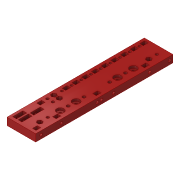
# Autodesk Inventor part: Coupler lift long
Saved by Autodesk Inventor 2020 (Build 240168000, 168)
## iProperties
Created: 2019-10-02
Part Number: Coupler lift long
Material: Generic
Document SubType Name: Modeling
Designer: ball
Density: 1 g/cm^3
Appearance: Default
Author: ball
Autodesk Inventor part; units mm, degrees
sketch "Sketch1" plane through (0, 0, 0) normal (0, 1, 0) x (-1, 0, 0)
  line L0 (0, 0) -> (35.5, 0)
  line L1 (35.5, 0) -> (35.5, -170)
  line L2 (35.5, -170) -> (0, -170)
  line L3 (0, -170) -> (0, 0)
  dimension "d0" = 35.5
  dimension "d1" = 170
  constraints: 8 end point, 2 parallel, 1 horizontal, 1 perpendicular
  measures "d0" distance of L1.end L2.end
  measures "d1" distance of L0.end L1.end
extrude "BlockShape" add sketch "Sketch1" along normal blind 9
sketch "Sketch2" plane through (0, 9, 0) normal (0, 1, 0) x (1, 0, 0)
  circle A0 centre (-10, 15) radius 3.25 construction
  line L0 (-35.5, 0) -> (0, 0) projected
  line L1 (0, 0) -> (0, 170) projected
  line L2 (-13.25, 15) -> (-11.625, 17.8146)
  line L3 (-11.625, 17.8146) -> (-8.375, 17.8146)
  line L4 (-8.375, 17.8146) -> (-6.75, 15)
  line L5 (-6.75, 15) -> (-8.375, 12.1854)
  line L6 (-8.375, 12.1854) -> (-11.625, 12.1854)
  line L7 (-11.625, 12.1854) -> (-13.25, 15)
  circle A1 centre (-10, 150) radius 3.25 construction
  line L8 (-13.25, 150) -> (-11.625, 152.8146)
  line L9 (-11.625, 152.8146) -> (-8.375, 152.8146)
  line L10 (-8.375, 152.8146) -> (-6.75, 150)
  line L11 (-6.75, 150) -> (-8.375, 147.1854)
  line L12 (-8.375, 147.1854) -> (-11.625, 147.1854)
  line L13 (-11.625, 147.1854) -> (-13.25, 150)
  line L14 (0, 170) -> (-35.5, 170) projected
  circle A2 centre (-10, 15) radius 1.7 construction
  circle A3 centre (-10, 150) radius 1.7 construction
  dimension "d7" = 6.5
  dimension "d10" = 6.5
  dimension "d23" = 135
  dimension "d24" = 15
  dimension "d25" = 10
  dimension "d28" = 3.4
  dimension "d29" = 3.4
  constraints: 24 end point, 4 coincident, 2 centre point, 2 horizontal alignment, 30 other
  measures "d23" distance of point (-10, 150) point (-10, 15)
  measures "d24" distance from line of L0 point (-10, 15)
  measures "d25" distance from line of L1 point (-10, 15)
  measures "d28" diameter of A2
  measures "d29" diameter of A3
extrude "SlideNutWell2" cut sketch "Sketch2" against normal blind 5
sketch "Sketch3" plane through (0, 0, 0) normal (0, -1, 0) x (1, 0, 0)
  circle A0 centre (-10, -25) radius 3.25 construction
  line L0 (0, 0) -> (-35.5, 0) projected
  line L1 (-35.5, 0) -> (-35.5, -170) projected
  line L2 (-11.6286, -27.8125) -> (-13.25, -24.9958)
  line L3 (-13.25, -24.9958) -> (-11.6214, -22.1833)
  line L4 (-11.6214, -22.1833) -> (-8.3714, -22.1875)
  line L5 (-8.3714, -22.1875) -> (-6.75, -25.0042)
  line L6 (-6.75, -25.0042) -> (-8.3786, -27.8167)
  line L7 (-8.3786, -27.8167) -> (-11.6286, -27.8125)
  circle A1 centre (-10, -160) radius 3.25 construction
  line L8 (-6.75, -160) -> (-8.375, -162.8146)
  line L9 (-8.375, -162.8146) -> (-11.625, -162.8146)
  line L10 (-11.625, -162.8146) -> (-13.25, -160)
  line L11 (-13.25, -160) -> (-11.625, -157.1854)
  line L12 (-11.625, -157.1854) -> (-8.375, -157.1854)
  line L13 (-8.375, -157.1854) -> (-6.75, -160)
  line L14 (0, -170) -> (0, 0) projected
  dimension "d15" = 6.5
  dimension "d18" = 6.5
  dimension "d16" = 25
  dimension "d19" = 135
  dimension "d26" = 10
  dimension "d27" = 10
  constraints: 24 end point, 2 coincident, 1 horizontal alignment, 31 other
  measures "d16" distance from line of L0 point (-10, -25)
  measures "d19" distance of point (-10, -160) point (-10, -25)
  measures "d26" distance from line of L14 point (-10, -25)
  measures "d27" distance from line of L14 point (-10, -160)
extrude "SlideNutWell1" cut sketch "Sketch3" against normal blind 5
sketch "Sketch5" plane through (0, 9, 0) normal (0, 1, 0) x (1, 0, 0)
  circle A0 centre (-10, 15) radius 1.7
  line L0 (0, 0) -> (0, 170) projected
  line L1 (-35.5, 0) -> (0, 0) projected
  circle A1 centre (-10, 150) radius 1.7
  circle A2 centre (-10, 25) radius 1.7
  circle A3 centre (-10, 160) radius 1.7
  dimension "d30" = 3.4
  dimension "d31" = 10
  dimension "d32" = 15
  dimension "d33" = 3.4
  dimension "d34" = 10
  dimension "d35" = 135
  dimension "d36" = 3.4
  dimension "d37" = 25
  dimension "d38" = 3.4
  dimension "d39" = 10
  dimension "d40" = 135
  constraints: 4 centre point
  measures "d30" diameter of A0
  measures "d31" distance from line of L0 A0.centre
  measures "d32" distance from line of L1 A0.centre
  measures "d33" diameter of A1
  measures "d34" distance from line of L0 A1.centre
  measures "d35" distance of A1.centre A0.centre
  measures "d36" diameter of A2
  measures "d37" distance from line of L1 A2.centre
  measures "d38" diameter of A3
  measures "d39" distance from line of L0 A3.centre
  measures "d40" distance of A2.centre A3.centre
extrude "SlideMoutingHoles" cut sketch "Sketch5" against normal through all
sketch "Sketch6" plane through (0, 9, 0) normal (0, 1, 0) x (1, 0, 0)
  line L0 (-32.5, 4) -> (-27.7502, 4)
  line L1 (-27.7502, 4) -> (-27.7502, 16.7)
  line L2 (-27.7502, 16.7) -> (-32.5, 16.7)
  line L3 (-32.5, 16.7) -> (-32.5, 4)
  line L4 (-35.5, 0) -> (0, 0) projected
  line L5 (-35.5, 170) -> (-35.5, 0) projected
  line L6 (-25.7502, 4) -> (-21.0002, 4)
  line L7 (-21.0002, 4) -> (-21.0002, 16.7)
  line L8 (-21.0002, 16.7) -> (-25.7502, 16.7)
  line L9 (-25.7502, 16.7) -> (-25.7502, 4)
  line L10 (0, 0) -> (0, 170) construction
  line L11 (-35.5, 170) -> (0, 170) projected
  line L12 (0, 0) -> (-20, 0) construction
  line L13 (-20, 0) -> (-20, 170) construction
  line L14 (-20, 170) -> (0, 170) construction
  line L15 (0, 170) -> (0, 0)
  circle A0 centre (-23.3752, 44.7) radius 1.7
  circle A1 centre (-30.125, 44.7) radius 1.7
  circle A2 centre (-30.125, 52.7) radius 1.7
  circle A3 centre (-23.3752, 52.7) radius 1.7
  line L16 (-25.7502, 18.7) -> (-21.0002, 18.7)
  line L17 (-21.0002, 18.7) -> (-21.0002, 31.4)
  line L18 (-21.0002, 31.4) -> (-25.7502, 31.4)
  line L19 (-25.7502, 31.4) -> (-25.7502, 18.7)
  dimension "d43" = 4.7498
  dimension "d44" = 12.7
  dimension "d45" = 4
  dimension "d46" = 3
  dimension "d47" = 4.75
  dimension "d48" = 2
  dimension "d49" = 20
  dimension "d50" = 3.4
  dimension "d51" = 28
  dimension "d87" = 3.4
  dimension "d88" = 5.375
  dimension "d90" = 3.4
  dimension "d91" = 8
  dimension "d92" = 3.4
  dimension "d180" = 4.75
  dimension "d181" = 12.7
  dimension "d182" = 2
  dimension "d183" = 12.7
  dimension "d184" = 4
  dimension "d260" = 28
  dimension "d261" = 8
  constraints: 32 end point, 8 parallel, 4 centre point, 4 horizontal, 4 perpendicular, 2 point on line
  measures "d43" distance of L2.end L1.end
  measures "d44" distance of L1.end L0.end
  measures "d45" distance between parallel lines of L4 L0
  measures "d46" distance between parallel lines of L5 L3
  measures "d47" distance of L8.end L7.end
  measures "d48" distance between parallel lines of L9 L1
  measures "d49" distance of L13.end L14.end
  measures "d50" diameter of A0
  measures "d51" distance from line of A0.centre L8
  measures "d87" diameter of A1
  measures "d88" distance from line of L5 A1.centre
  measures "d90" diameter of A2
  measures "d91" distance of A2.centre A1.centre
  measures "d92" diameter of A3
  measures "d180" distance of L18.end L17.end
  measures "d181" distance of L17.end L16.end
  measures "d182" distance between parallel lines of L16 L8
  measures "d183" distance between parallel lines of L8 L6
  measures "d184" distance between parallel lines of L4 L6
  measures "d260" distance from line of L2 A1.centre
  measures "d261" distance of A0.centre A3.centre
extrude "PulleyHoles" cut sketch "Sketch6" against normal through all contours L3 L2 L1 L0 | L9 L8 L7 L6 | A0 | A1 | A2 | A3 | L19 L18 L17 L16
sketch "Sketch7" plane through (0, 0, 0) normal (0, -1, 0) x (1, 0, 0)
  circle A0 centre (-23.3752, -44.7) radius 1.7 projected
  circle A1 centre (-23.3752, -44.7) radius 3.25 construction
  circle A2 centre (-30.1625, -44.7) radius 3.25 construction
  line L0 (-30.125, -41.4502) -> (-27.3294, -43.1076)
  line L1 (-27.3294, -43.1076) -> (-27.3669, -46.3574)
  line L2 (-27.3669, -46.3574) -> (-30.2, -47.9498)
  line L3 (-30.2, -47.9498) -> (-32.9956, -46.2924)
  line L4 (-32.9956, -46.2924) -> (-32.9581, -43.0426)
  line L5 (-32.9581, -43.0426) -> (-30.125, -41.4502)
  circle A3 centre (-30.125, -44.7) radius 1.7 projected
  line L6 (-20.1252, -44.7) -> (-21.7502, -47.5146)
  line L7 (-21.7502, -47.5146) -> (-25.0002, -47.5146)
  line L8 (-25.0002, -47.5146) -> (-26.6252, -44.7)
  line L9 (-26.6252, -44.7) -> (-25.0002, -41.8854)
  line L10 (-25.0002, -41.8854) -> (-21.7502, -41.8854)
  line L11 (-21.7502, -41.8854) -> (-20.1252, -44.7)
  point P0 (0, 0)
  dimension "d54" = 6.5
  dimension "d89" = 6.5
  dimension "d262" = 0
  constraints: 24 end point, 4 coincident, 1 horizontal alignment, 32 other
  measures "d262" vertical distance of point (-30.162, -44.7) A3.centre
extrude "TensionNutWells2" cut sketch "Sketch7" against normal blind 5 contours A0 | L0 L1 L2 L3 L4 L5 | A3 | L6 L7 L8 L9 L10 L11
sketch "Sketch8" plane through (-35.5, 0, -170) normal (-1, 0, 0) x (0, 0, 1)
  circle A0 centre (159.65, 4.5) radius 1.4605
  line L0 (0, 9) -> (170, 9) projected
  line L1 (170, 0) -> (170, 9) projected
  circle A1 centre (144.95, 4.5) radius 1.45
  dimension "d57" = 2.921
  dimension "d58" = 4.5
  dimension "d59" = 10.35
  dimension "d185" = 2.9
  dimension "d186" = 14.7
  dimension "d187" = 4.5
  constraints: 2 centre point
  measures "d57" diameter of A0
  measures "d58" distance from line of L0 A0.centre
  measures "d59" distance from line of L1 A0.centre
  measures "d185" diameter of A1
  measures "d186" distance of A1.centre A0.centre
  measures "d187" distance from line of L0 A1.centre
hole "PulleyMountingHole" at (-35.5, 4.5, -10.35) at (-35.5, 4.5, -25.05) direction (1, 0, 0) diameter 2.921 depth 21 counterbore diameter 3.4 counterbore depth 1.5
sketch "Sketch9" plane through (-21.0002, 9, -16.7) normal (-1, 0, 0) x (0, 0, 1)
  circle A0 centre (6.35, -4.5) radius 1.4605 projected
  circle A1 centre (6.35, -4.5) radius 2.54
  circle A2 centre (-8.35, -4.5) radius 1.4605 projected
  circle A3 centre (-8.35, -4.5) radius 2.54
  point P0 (16.7, -9)
  dimension "d67" = 5.08
  dimension "d194" = 5.08
  constraints: 2 centre point, 2 coincident
  measures "d67" diameter of A1
  measures "d194" diameter of A3
extrude "PulleyStandoff4" add sketch "Sketch9" along normal blind 0.2032
sketch "Sketch11" plane through (-25.7502, 9, -4) normal (1, 0, 0) x (0, 0, -1)
  circle A0 centre (6.35, -4.5) radius 2.54
  circle A1 centre (6.35, -4.5) radius 1.4605
  circle A2 centre (21.05, -4.5) radius 1.4605 projected
  circle A3 centre (21.05, -4.5) radius 2.54
  point P0 (-4, -9)
  dimension "d73" = 5.08
  dimension "d195" = 5.08
  constraints: 3 centre point, 3 coincident
  measures "d73" diameter of A0
  measures "d195" diameter of A3
sketch "Sketch12" plane through (-32.5, 9, -4) normal (1, 0, 0) x (0, 0, -1)
  circle A0 centre (6.35, -4.5) radius 2.54
  circle A1 centre (6.35, -4.5) radius 1.4605
  point P0 (-4, -9)
  dimension "d76" = 5.08
  constraints: 2 centre point, 1 coincident
  measures "d76" diameter of A0
extrude "PulleyStandoff1" add sketch "Sketch12" along normal blind 0.2032
sketch "Sketch10" plane through (-27.7502, 9, -16.7) normal (-1, 0, 0) x (0, 0, 1)
  circle A0 centre (6.35, -4.5) radius 2.54
  circle A1 centre (6.35, -4.5) radius 1.4605
  point P0 (16.7, -9)
  dimension "d70" = 5.08
  constraints: 2 centre point, 2 coincident
  measures "d70" diameter of A0
extrude "PulleyStandoff2" add sketch "Sketch10" along normal blind 0.2032
extrude "PulleyStandoff3" add sketch "Sketch11" along normal blind 0.2032
sketch "Sketch14" plane through (0, 0, -170) normal (0, 0, -1) x (-1, 0, 0)
  circle A0 centre (18, 4.5) radius 2.25
  line L0 (35.5, 0) -> (0, 0) projected
  line L1 (0, 0) -> (0, 9) projected
  dimension "d82" = 4.5
  dimension "d83" = 4.5
  dimension "d84" = 18
  constraints: 1 centre point
  measures "d82" diameter of A0
  measures "d83" distance from line of L0 A0.centre
  measures "d84" distance from line of L1 A0.centre
extrude "4mmShaftHole" cut sketch "Sketch14" against normal blind 71
sketch "Sketch15" plane through (0, 9, 0) normal (0, 1, 0) x (1, 0, 0)
  circle A0 centre (-30.125, 52.7) radius 1.7 projected
  circle A1 centre (-30.125, 52.7) radius 3.25 construction
  circle A2 centre (-23.3752, 52.7) radius 1.7 projected
  circle A3 centre (-23.3752, 52.7) radius 3.25 construction
  line L0 (-30.125, 49.45) -> (-32.9396, 51.075)
  line L1 (-32.9396, 51.075) -> (-32.9396, 54.325)
  line L2 (-32.9396, 54.325) -> (-30.125, 55.95)
  line L3 (-30.125, 55.95) -> (-27.3104, 54.325)
  line L4 (-27.3104, 54.325) -> (-27.3104, 51.075)
  line L5 (-27.3104, 51.075) -> (-30.125, 49.45)
  line L6 (-23.3752, 49.45) -> (-26.1898, 51.075)
  line L7 (-26.1898, 51.075) -> (-26.1898, 54.325)
  line L8 (-26.1898, 54.325) -> (-23.3752, 55.95)
  line L9 (-23.3752, 55.95) -> (-20.5606, 54.325)
  line L10 (-20.5606, 54.325) -> (-20.5606, 51.075)
  line L11 (-20.5606, 51.075) -> (-23.3752, 49.45)
  point P0 (0, 0)
  dimension "d93" = 6.5
  dimension "d94" = 6.5
  constraints: 24 end point, 4 coincident, 2 vertical alignment, 30 other
extrude "TensionNutWells1" cut sketch "Sketch15" against normal blind 5
ref_plane "PulleyMidPlane1" through (-30.1251, 9, -4) normal (1, 0, 0) x (0, 0, -1)
ref_plane "PulleyMidPlane2" through (-23.3752, 9, -16.7) normal (-1, 0, 0) x (0, 0, 1)
sketch "Sketch16" plane through (0, 9, 0) normal (0, 1, 0) x (1, 0, 0)
  circle A0 centre (-9.525, 40) radius 1.9304 construction
  line L0 (0, 0) -> (0, 170) construction
  circle A1 centre (-10, 25) radius 1.7 construction
  circle A2 centre (-9.525, 59.558) radius 1.9304 construction
  circle A3 centre (-9.525, 130.442) radius 1.9304 construction
  circle A4 centre (-10, 150) radius 1.7 construction
  circle A5 centre (-9.525, 110.884) radius 1.9304 construction
  dimension "d97" = 3.8608
  dimension "d98" = 9.525
  dimension "d99" = 15
  dimension "d100" = 3.8608
  dimension "d101" = 19.558
  dimension "d102" = 3.8608
  dimension "d103" = 9.525
  dimension "d104" = 19.558
  dimension "d105" = 3.8608
  dimension "d106" = 19.558
  constraints: 4 centre point
  measures "d97" diameter of A0
  measures "d98" distance from line of L0 A0.centre
  measures "d99" vertical distance of A1.centre A0.centre
  measures "d100" diameter of A2
  measures "d101" distance of A2.centre A0.centre
  measures "d102" diameter of A3
  measures "d103" distance from line of L0 A3.centre
  measures "d104" vertical distance of A4.centre A3.centre
  measures "d105" diameter of A5
  measures "d106" distance of A3.centre A5.centre
hole "XRailMoutingHoles1" at (-9.525, 9, -40) at (-9.525, 9, -59.558) at (-9.525, 9, -110.884) at (-9.525, 9, -130.442) direction (0, -1, 0) diameter 3.8608 end through all counterbore diameter 8.89 counterbore depth 3.048
sketch "Sketch17" plane through (0, 0, 0) normal (0, -1, 0) x (1, 0, 0)
  circle A0 centre (-9.525, -120.663) radius 1.9304 construction
  circle A1 centre (-9.525, -130.442) radius 1.9304 projected
  circle A2 centre (-9.525, -101.105) radius 1.9304 construction
  circle A3 centre (-9.525, -49.779) radius 1.9304 construction
  circle A4 centre (-9.525, -69.337) radius 1.9304 construction
  circle A5 centre (-9.525, -40) radius 1.9304 construction
  point P0 (0, 0)
  dimension "d114" = 3.8608
  dimension "d115" = 9.779
  dimension "d116" = 3.8608
  dimension "d117" = 19.558
  dimension "d118" = 3.8608
  dimension "d119" = 3.8608
  dimension "d120" = 9.779
  dimension "d121" = 19.558
  constraints: 4 centre point
  measures "d114" diameter of A0
  measures "d115" distance of A0.centre A1.centre
  measures "d116" diameter of A2
  measures "d117" distance of A2.centre A0.centre
  measures "d118" diameter of A3
  measures "d119" diameter of A4
  measures "d120" distance of A3.centre A5.centre
  measures "d121" distance of A4.centre A3.centre
hole "XRailMoutingHoles2" at (-9.525, 0, -120.663) at (-9.525, 0, -101.105) at (-9.525, 0, -69.337) at (-9.525, 0, -49.779) direction (0, 1, 0) diameter 3.8608 end through all counterbore diameter 8.89 counterbore depth 3.048
sketch "Sketch19" plane through (0, 0, 0) normal (1, 0, 0) x (0, 0, -1)
  line L0 (12.1854, 9) -> (12.1854, 4) construction
  line L1 (67.4066, 9) -> (71.2674, 9) construction
  line L2 (99.1746, 9) -> (103.0354, 9) construction
  line L3 (125.997, 9) -> (134.887, 9) construction
  line L4 (147.1854, 9) -> (147.1854, 4) construction
  line L5 (158.3, 9) -> (161.7, 9) construction
  line L6 (170, 0) -> (0, 0) projected
  line L7 (0, 0) -> (0, 9) projected
  circle A0 centre (76.2674, 4.5) radius 1.7
  circle A1 centre (86.2674, 4.5) radius 1.7
  circle A2 centre (96.2674, 4.5) radius 1.7
  line L8 (170, 0) -> (170, 9) projected
  circle A3 centre (165.85, 4.5) radius 1.7
  dimension "d159" = 27.9072
  dimension "d160" = 3.4
  dimension "d161" = 4.5
  dimension "d162" = 5
  dimension "d165" = 10
  dimension "d170" = 8.3
  dimension "d171" = 3.4
  dimension "d172" = 4.5
  dimension "d173" = 4.15
  dimension "d174" = 12.2984
  constraints: 4 centre point, 1 horizontal, 4 other
  measures "d159" distance of L1.end L2.start
  measures "d160" diameter of A0
  measures "d161" distance from line of L6 A0.centre
  measures "d162" horizontal distance of L1.end A0.centre
  measures "d165" distance of A0.centre A1.centre
  measures "d170" distance from line of L8 L5.end
  measures "d171" diameter of A3
  measures "d172" distance from line of L6 A3.centre
  measures "d173" distance from line of L8 A3.centre
  measures "d174" distance from line of L3.end L4
extrude "NonPulleySideHoles" cut sketch "Sketch19" against normal blind 13 contours A0 | A2 | A3
ref_plane "Work Plane3" through (-7.7, 0, 0) normal (1, 0, 0) x (0, 0, -1)
sketch "Sketch20" plane through (-7.7, 0, 0) normal (1, 0, 0) x (0, 0, -1)
  circle A0 centre (6.65, 4.5) radius 3.45 construction
  line L0 (0, 0) -> (0, 9) construction
  line L1 (0, 0) -> (170, 0) construction
  line L2 (6.65, 1.05) -> (3.6622, 2.775)
  line L3 (3.6622, 2.775) -> (3.6622, 9)
  line L4 (9.6378, 9) -> (9.6378, 2.775)
  line L5 (9.6378, 2.775) -> (6.65, 1.05)
  line L6 (170, 9) -> (0, 9) projected
  line L7 (3.6622, 9) -> (9.6378, 9)
  circle A1 centre (96.2674, 4.5) radius 1.7 projected
  circle A2 centre (76.2674, 4.5) radius 1.7 projected
  circle A3 centre (81.2674, 4.5) radius 3.45 construction
  line L8 (81.2674, 1.05) -> (78.2796, 2.775)
  line L9 (78.2796, 2.775) -> (78.2796, 9)
  line L10 (84.2552, 9) -> (84.2552, 2.775)
  line L11 (84.2552, 2.775) -> (81.2674, 1.05)
  line L12 (78.2796, 9) -> (84.2552, 9)
  line L13 (147.1854, 9) -> (147.1854, 4) construction
  line L14 (134.887, 5.952) -> (134.887, 9) construction
  circle A4 centre (141.0362, 4.5) radius 3.45 construction
  line L15 (141.0362, 1.05) -> (138.0484, 2.775)
  line L16 (138.0484, 2.775) -> (138.0484, 9)
  line L17 (144.024, 9) -> (144.024, 2.775)
  line L18 (144.024, 2.775) -> (141.0362, 1.05)
  line L19 (138.0484, 9) -> (144.024, 9)
  circle A5 centre (31.6858, 4.5) radius 3.45 construction
  circle A6 centre (31.6858, 4.5) radius 3.45 construction
  line L20 (31.6858, 1.05) -> (28.698, 2.775)
  line L21 (28.698, 2.775) -> (28.698, 9)
  line L22 (34.6736, 9) -> (34.6736, 2.775)
  line L23 (34.6736, 2.775) -> (31.6858, 1.05)
  line L24 (28.698, 9) -> (34.6736, 9)
  point P0 (86.2674, 4.5)
  dimension "d199" = 6.9
  dimension "d204" = 6.9
  dimension "d207" = 6.9
  dimension "d279" = 6.9
  dimension "d200" = 6.65
  dimension "d201" = 4.5
  dimension "d202" = 20
  dimension "d203" = 10
  dimension "d205" = 12.2984
  dimension "d206" = 6.1492
  dimension "d276" = 6.9
  dimension "d277" = 31.6858
  dimension "d278" = 4.5
  constraints: 40 end point, 4 coincident, 4 vertical alignment, 2 point on line, 1 centre point, 32 other
  measures "d200" distance from line of L0 point (6.65, 4.5)
  measures "d201" distance from line of L1 point (6.65, 4.5)
  measures "d202" distance of A1.centre A2.centre
  measures "d203" distance of A2.centre point (86.267, 4.5)
  measures "d205" distance between parallel lines of L13 L14
  measures "d206" distance from line of point (141.036, 4.5) L14
  measures "d276" diameter of A5
  measures "d277" distance from line of L0 A5.centre
  measures "d278" distance from line of L1 A5.centre
extrude "SideNutWellsNonPulleySide" cut sketch "Sketch20" along normal blind 4.4 contours L6 L17 L18 L15 L16 | L6 L10 L11 L8 L9 | L6 L22 L23 L20 L21 | L2 L3 L6 L4 L5
sketch "Sketch21" plane through (0, 0, 0) normal (1, 0, 0) x (0, 0, -1)
  line L0 (3.6622, 9) -> (3.6622, 2.775) construction
  line L1 (9.6378, 2.775) -> (9.6378, 9) construction
  line L2 (78.2796, 9) -> (78.2796, 2.775) construction
  line L3 (84.2552, 2.775) -> (84.2552, 9) construction
  line L4 (138.0484, 9) -> (138.0484, 2.775) construction
  line L5 (144.024, 2.775) -> (144.024, 9) construction
  circle A0 centre (6.65, 4.5) radius 1.7
  line L6 (170, 0) -> (0, 0) projected
  circle A1 centre (81.2674, 4.5) radius 1.7
  circle A2 centre (141.0362, 4.5) radius 1.7
  line L7 (27.8167, 0) -> (27.8167, 5) construction
  line L8 (35.555, 5.952) -> (35.555, 9) construction
  circle A3 centre (31.6858, 4.5) radius 1.7
  line L9 (0, 0) -> (0, 9) projected
  dimension "d210" = 3.4
  dimension "d211" = 5.9756
  dimension "d212" = 2.9878
  dimension "d213" = 4.5
  dimension "d214" = 3.4
  dimension "d215" = 2.9878
  dimension "d216" = 5.9756
  dimension "d217" = 4.5
  dimension "d218" = 5.9756
  dimension "d219" = 3.4
  dimension "d220" = 2.9878
  dimension "d221" = 4.5
  dimension "d271" = 7.7383
  dimension "d272" = 3.4
  dimension "d273" = 3.8692
  dimension "d274" = 4.5
  dimension "d275" = 31.6858
  constraints: 4 centre point
  measures "d210" diameter of A0
  measures "d211" distance between parallel lines of L1 L0
  measures "d212" distance from line of L0 A0.centre
  measures "d213" distance from line of L6 A0.centre
  measures "d214" diameter of A1
  measures "d215" distance from line of L2 A1.centre
  measures "d216" distance between parallel lines of L3 L2
  measures "d217" distance from line of L6 A1.centre
  measures "d218" distance between parallel lines of L5 L4
  measures "d219" diameter of A2
  measures "d220" distance from line of L4 A2.centre
  measures "d221" distance from line of L6 A2.centre
  measures "d271" distance between parallel lines of L7 L8
  measures "d272" diameter of A3
  measures "d273" distance from line of A3.centre L8
  measures "d274" distance from line of L6 A3.centre
  measures "d275" distance from line of L9 A3.centre
extrude "SideNutWellHolesNonPulleySide" cut sketch "Sketch21" against normal blind 8.4
ref_plane "Work Plane4" through (-27.8, 0, -170) normal (-1, 0, 0) x (0, 0, 1)
sketch "Sketch22" plane through (-35.5, 0, -170) normal (-1, 0, 0) x (0, 0, 1)
  line L0 (170, 0) -> (0, 0) projected
  line L1 (0, 9) -> (170, 9) projected
  circle A0 centre (6, 4.5) radius 1.7
  line L2 (0, 0) -> (0, 9) projected
  circle A1 centre (18, 4.5) radius 1.7
  circle A2 centre (30, 4.5) radius 1.7
  circle A3 centre (42, 4.5) radius 1.7
  circle A4 centre (54, 4.5) radius 1.7
  circle A5 centre (66, 4.5) radius 1.7
  circle A6 centre (78, 4.5) radius 1.7
  circle A7 centre (90, 4.5) radius 1.7
  circle A8 centre (102, 4.5) radius 1.7
  line L3 (138.6, 9) -> (138.6, 0) construction
  line L4 (128.5498, 0) -> (128.5498, 5) construction
  circle A9 centre (133.5749, 4.5) radius 1.7
  dimension "d225" = 9
  dimension "d226" = 3.4
  dimension "d227" = 6
  dimension "d228" = 4.5
  dimension "d231" = 12
  dimension "d263" = 3.4
  dimension "d264" = 4.5
  dimension "d265" = 10.0502
  dimension "d266" = 5.0251
  constraints: 10 centre point, 1 horizontal, 16 other
  measures "d225" distance between parallel lines of L0 L1
  measures "d226" diameter of A0
  measures "d227" distance from line of L2 A0.centre
  measures "d228" distance from line of L0 A0.centre
  measures "d231" distance of A0.centre A1.centre
  measures "d263" diameter of A9
  measures "d264" distance from line of L0 A9.centre
  measures "d265" distance between parallel lines of L3 L4
  measures "d266" distance from line of L4 A9.centre
extrude "NutWellHolesPulleySide" cut sketch "Sketch22" against normal blind 8.4
sketch "Sketch23" plane through (-27.8, 0, -170) normal (-1, 0, 0) x (0, 0, 1)
  circle A0 centre (6, 4.5) radius 1.7 construction
  circle A1 centre (6, 4.5) radius 3.45 construction
  line L0 (6, 1.05) -> (3.0122, 2.775)
  line L1 (3.0122, 2.775) -> (3.0122, 9)
  line L2 (8.9878, 9) -> (8.9878, 2.775)
  line L3 (8.9878, 2.775) -> (6, 1.05)
  line L4 (170, 9) -> (0, 9) projected
  line L5 (3.0122, 9) -> (8.9878, 9)
  circle A2 centre (18, 4.5) radius 3.45 construction
  line L6 (18, 1.05) -> (15.0122, 2.775)
  line L7 (15.0122, 2.775) -> (15.0122, 9)
  line L8 (20.9878, 9) -> (20.9878, 2.775)
  line L9 (20.9878, 2.775) -> (18, 1.05)
  line L10 (15.0122, 9) -> (20.9878, 9)
  circle A3 centre (30, 4.5) radius 3.45 construction
  line L11 (30, 1.05) -> (27.0122, 2.775)
  line L12 (27.0122, 2.775) -> (27.0122, 9)
  line L13 (32.9878, 9) -> (32.9878, 2.775)
  line L14 (32.9878, 2.775) -> (30, 1.05)
  line L15 (27.0122, 9) -> (32.9878, 9)
  circle A4 centre (42, 4.5) radius 3.45 construction
  line L16 (42, 1.05) -> (39.0122, 2.775)
  line L17 (39.0122, 2.775) -> (39.0122, 9)
  line L18 (44.9878, 9) -> (44.9878, 2.775)
  line L19 (44.9878, 2.775) -> (42, 1.05)
  line L20 (39.0122, 9) -> (44.9878, 9)
  circle A5 centre (54, 4.5) radius 3.45 construction
  line L21 (54, 1.05) -> (51.0122, 2.775)
  line L22 (51.0122, 2.775) -> (51.0122, 9)
  line L23 (56.9878, 9) -> (56.9878, 2.775)
  line L24 (56.9878, 2.775) -> (54, 1.05)
  line L25 (51.0122, 9) -> (56.9878, 9)
  circle A6 centre (66, 4.5) radius 3.45 construction
  line L26 (66, 1.05) -> (63.0122, 2.775)
  line L27 (63.0122, 2.775) -> (63.0122, 9)
  line L28 (68.9878, 9) -> (68.9878, 2.775)
  line L29 (68.9878, 2.775) -> (66, 1.05)
  line L30 (63.0122, 9) -> (68.9878, 9)
  circle A7 centre (78, 4.5) radius 3.45 construction
  line L31 (78, 1.05) -> (75.0122, 2.775)
  line L32 (75.0122, 2.775) -> (75.0122, 9)
  line L33 (80.9878, 9) -> (80.9878, 2.775)
  line L34 (80.9878, 2.775) -> (78, 1.05)
  line L35 (75.0122, 9) -> (80.9878, 9)
  circle A8 centre (90, 4.5) radius 3.45 construction
  line L36 (90, 1.05) -> (87.0122, 2.775)
  line L37 (87.0122, 2.775) -> (87.0122, 9)
  line L38 (92.9878, 9) -> (92.9878, 2.775)
  line L39 (92.9878, 2.775) -> (90, 1.05)
  line L40 (87.0122, 9) -> (92.9878, 9)
  circle A9 centre (102, 4.5) radius 3.45 construction
  line L41 (102, 1.05) -> (99.0122, 2.775)
  line L42 (99.0122, 2.775) -> (99.0122, 9)
  line L43 (104.9878, 9) -> (104.9878, 2.775)
  line L44 (104.9878, 2.775) -> (102, 1.05)
  line L45 (99.0122, 9) -> (104.9878, 9)
  circle A10 centre (133.5749, 4.5) radius 1.7 construction
  circle A11 centre (133.5749, 4.5) radius 3.45 construction
  line L46 (133.5749, 1.05) -> (130.5871, 2.775)
  line L47 (130.5871, 2.775) -> (130.5871, 9)
  line L48 (136.5627, 9) -> (136.5627, 2.775)
  line L49 (136.5627, 2.775) -> (133.5749, 1.05)
  line L50 (130.5871, 9) -> (136.5627, 9)
  point P0 (170, 0)
  point P1 (75.0122, 9)
  point P2 (68.9878, 9)
  point P3 (51.0122, 9)
  point P4 (44.9878, 9)
  point P5 (27.0122, 9)
  point P6 (20.9878, 9)
  point P7 (15.0122, 9)
  dimension "d238" = 6.9
  dimension "d241" = 12
  constraints: 100 end point, 64 horizontal alignment, 32 parallel, 20 coincident, 10 vertical alignment, 8 collinear, 29 other
  measures "d241" distance of point (6, 4.5) point (18, 4.5)
extrude "NutWellsPulleySide" cut sketch "Sketch23" along normal blind 4.4
sketch "Sketch24" plane through (0, 9, 0) normal (0, 1, 0) x (1, 0, 0)
  circle A0 centre (-29.5, 158) radius 1.524
  line L0 (0, 170) -> (-35.5, 170) projected
  line L1 (-35.5, 170) -> (-35.5, 0) projected
  circle A1 centre (-29.5, 146) radius 1.524
  circle A2 centre (-29.5, 134) radius 1.524
  circle A3 centre (-29.5, 122) radius 1.524
  circle A4 centre (-29.5, 110) radius 1.524
  circle A5 centre (-29.5, 98) radius 1.524
  circle A6 centre (-29.5, 86) radius 1.524
  circle A7 centre (-29.5, 74) radius 1.524
  circle A8 centre (-29.5, 62) radius 1.524
  point P0 (0, 0)
  dimension "d248" = 3.048
  dimension "d249" = 12
  dimension "d250" = 6
  dimension "d253" = 12
  constraints: 9 centre point, 1 vertical, 16 other
  measures "d248" diameter of A0
  measures "d249" distance from line of L0 A0.centre
  measures "d250" distance from line of L1 A0.centre
  measures "d253" distance of A0.centre A1.centre
extrude "TieWrapHoles" cut sketch "Sketch24" against normal through all
equation "\"d183\" = d44"
equation "\"d184\" = d45"
equation "\"d260\" = d51"
equation "\"d261\" = d91"
equation "\"d187\" = d58"
equation "\"d103\" = d98"
equation "\"d104\" = d101"
equation "\"d106\" = d101"
equation "\"d115\" = 0.5 * d101"
equation "\"d117\" = d101"
equation "\"d120\" = d115"
equation "\"d121\" = d101"
equation "\"d161\" = d156"
equation "\"d172\" = d156"
equation "\"d173\" = 0.5 * d170"
equation "\"d203\" = 0.5 * d202"
equation "\"d206\" = 0.5 * d205"
equation "\"d277\" = d275"
equation "\"d278\" = d201"
equation "\"d212\" = 0.5 * d211"
equation "\"d215\" = 0.5 * d216"
equation "\"d217\" = d213"
equation "\"d220\" = 0.5 * d218"
equation "\"d221\" = d217"
equation "\"d273\" = 0.5 * d271"
equation "\"d274\" = d213"
equation "\"d228\" = 0.5 * d225"
equation "\"d264\" = d228"
equation "\"d266\" = 0.5 * d265"
equation "\"d135\" = 0.5 * d131"
equation "\"d156\" = d135"
equation "\"d131\" = 9"
body "Solid1"
